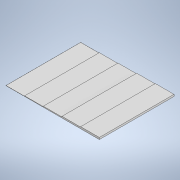
# Autodesk Inventor part: trap voor licht
Saved by Autodesk Inventor 2021 (Build 250183000, 183)
## iProperties
Created: 2023-10-23
Part Number: trap voor licht
Material: Generic
Document SubType Name: Modeling
Designer: Elias
Density: 1 g/cm^3
Appearance: Default
Author: Elias
Autodesk Inventor part; units mm, degrees
ref_plane "YZ Plane" through (0, 0, 0) normal (1, 0, 0) x (0, 1, 0)
ref_plane "XZ Plane" through (0, 0, 0) normal (0, 1, 0) x (-1, 0, 0)
ref_plane "XY Plane" through (0, 0, 0) normal (0, 0, 1) x (1, 0, 0)
sketch "Sketch1" plane through (0, 0, 0) normal (0, 0, 1) x (1, 0, 0)
  line L0 (0, 0) -> (50, 0)
  line L1 (0, 0) -> (0, 0.1)
  line L2 (0, 0.1) -> (10, 0.1)
  line L3 (10, 0.1) -> (10, 0.3)
  line L4 (10, 0.3) -> (20, 0.3)
  line L5 (20, 0.3) -> (20, 0.5)
  line L6 (20, 0.5) -> (30, 0.5)
  line L7 (30, 0.5) -> (30, 0.8)
  line L8 (30, 0.8) -> (40, 0.8)
  line L9 (40, 0.8) -> (40, 1)
  line L10 (40, 1) -> (50, 1)
  line L11 (50, 1) -> (50, 0)
  dimension "d3" = 0.1
  dimension "d4" = 10
  dimension "d5" = 0.2
  dimension "d6" = 10
  dimension "d7" = 0.2
  dimension "d8" = 10
  dimension "d9" = 0.3
  dimension "d10" = 10
  dimension "d11" = 0.2
  constraints: 24 end point, 6 perpendicular, 3 vertical, 1 horizontal, 1 parallel
  measures "d3" distance of L0.start L1.end
  measures "d4" distance of L1.end L2.end
  measures "d5" distance of L2.end L3.end
  measures "d6" distance of L3.end L4.end
  measures "d7" distance of L4.end L5.end
  measures "d8" distance of L5.end L6.end
  measures "d9" distance of L6.end L7.end
  measures "d10" distance of L7.end L8.end
  measures "d11" distance of L8.end L9.end
extrude "Extrusion1" add sketch "Sketch1" along normal blind 40
body "Solid1"
